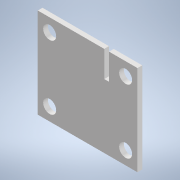
# Autodesk Inventor part: Part12
Saved by Autodesk Inventor 2020.2 (Build 242310000, 310)
## iProperties
Created: 2022-11-15
Part Number: Part12
Material: 一般
Document SubType Name: Modeling
Designer: Administrator
Density: 1 g/cm^3
Appearance: 既定
Author: Administrator
Autodesk Inventor part; units mm, degrees
ref_plane "YZ Plane" through (0, 0, 0) normal (1, 0, 0) x (0, 1, 0)
ref_plane "XZ Plane" through (0, 0, 0) normal (0, 1, 0) x (-1, 0, 0)
ref_plane "XY Plane" through (0, 0, 0) normal (0, 0, 1) x (1, 0, 0)
sketch "スケッチ1" plane through (0, 0, 0) normal (0, 0, 1) x (1, 0, 0)
  circle A0 centre (5, 0) radius 2.75 projected
  line L0 (14, -5.5) -> (14, 5.5) projected
  line L1 (0, 5.5) -> (14, 5.5) projected
  line L2 (0, -5.5) -> (0, 5.5) projected
  line L3 (14, -5.5) -> (0, -5.5) projected
  circle A1 centre (5, 27) radius 2.75 projected
  line L4 (14, 21.5) -> (14, 32.5) projected
  line L5 (0, 32.5) -> (14, 32.5) projected
  line L6 (0, 21.5) -> (0, 32.5) projected
  line L7 (14, 21.5) -> (0, 21.5) projected
  line L8 (30, 21.5) -> (30, 32.5) projected
  circle A2 centre (37, 27) radius 2.75 projected
  line L9 (42, 21.5) -> (42, 32.5) projected
  line L10 (28, 32.5) -> (42, 32.5) projected
  line L11 (28, 21.5) -> (28, 32.5) projected
  line L12 (42, 21.5) -> (28, 21.5) projected
  circle A3 centre (37, 0) radius 2.75 projected
  line L13 (42, -5.5) -> (42, 5.5) projected
  line L14 (28, 5.5) -> (42, 5.5) projected
  line L15 (28, -5.5) -> (28, 5.5) projected
  line L16 (42, -5.5) -> (28, -5.5) projected
  line L17 (0, -5.5) -> (42, -5.5)
  line L18 (42, -5.5) -> (42, 32.5)
  line L19 (42, 32.5) -> (0, 32.5)
  line L20 (0, 32.5) -> (0, -5.5)
  point P0 (0, 0)
  constraints: 8 end point, 2 parallel, 1 horizontal, 1 perpendicular
extrude "押し出し1" add sketch "スケッチ1" along normal blind 2 contours L3 L2 L1 L0 | L0 L1 L20 L7 L4 L19 L11 L12 L18 L14 L15 L17 | L15 L14 L13 L16 | L6 L5 L4 L7 | L12 L8 L10 L9
